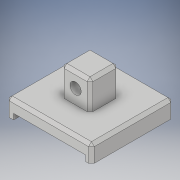
# Autodesk Inventor part: Raspberrycamhalter
Saved by Autodesk Inventor 2018.3 (Build 223284000, 284)
## iProperties
Part Number: Raspberrycamhalter
Material: Generisch
Document SubType Name: Modeling
Designer: pgmadmin
Density: 1 g/cm^3
Appearance: Vorgabe
Author: pgmadmin
Autodesk Inventor part; units mm, degrees
ref_plane "YZ Plane" through (0, 0, 0) normal (1, 0, 0) x (0, 1, 0)
ref_plane "XZ Plane" through (0, 0, 0) normal (0, 1, 0) x (-1, 0, 0)
ref_plane "XY Plane" through (0, 0, 0) normal (0, 0, 1) x (1, 0, 0)
sketch "Skizze1" plane through (0, 0, 0) normal (0, 0, 1) x (1, 0, 0)
  point P0 (0, 0)
sketch "Skizze2" plane through (0, 0, 0) normal (0, 0, 1) x (1, 0, 0)
  line L0 (-12.75, 12.25) -> (12.75, 12.25)
  line L1 (12.75, 12.25) -> (12.75, -12.25)
  line L2 (12.75, -12.25) -> (-12.75, -12.25)
  line L3 (-12.75, -12.25) -> (-12.75, 12.25)
  line L4 (0, 19.95) -> (0, -19.95) projected
  line L5 (-20.65, 0) -> (20.65, 0) projected
  line L6 (-14.75, 14.25) -> (14.75, 14.25)
  line L7 (14.75, 14.25) -> (14.75, -14.25)
  line L8 (14.75, -14.25) -> (-14.75, -14.25)
  line L9 (-14.75, -14.25) -> (-14.75, 14.25)
  point P0 (0, 0)
  dimension "d0" = 25.5
  dimension "d1" = 24.5
  dimension "d2" = 2
  dimension "d3" = 2
  dimension "d4" = 2
  dimension "d5" = 2
  constraints: 16 end point, 4 parallel, 2 horizontal, 2 perpendicular, 2 other
  measures "d0" distance of L1.end L2.end
  measures "d1" distance of L0.end L1.end
  measures "d2" distance between parallel lines of L6 L0
  measures "d3" distance between parallel lines of L3 L9
  measures "d4" distance between parallel lines of L2 L8
  measures "d5" distance between parallel lines of L7 L1
extrude "Extrusion1" add sketch "Skizze2" along normal blind 4 contours L3 L5 L9 L6 L4 L0 | L4 L6 L7 L5 L1 L0 | L3 L2 L4 L8 L9 L5 | L5 L7 L8 L4 L2 L1
sketch "Skizze3" plane through (0, 0, 4) normal (0, 0, 1) x (1, 0, 0)
  line L0 (14.75, -14.25) -> (-14.75, -14.25) projected
  line L1 (-14.75, 14.25) -> (14.75, 14.25)
  line L2 (14.75, 14.25) -> (14.75, -14.25)
  line L3 (14.75, -14.25) -> (-14.75, -14.25)
  line L4 (-14.75, -14.25) -> (-14.75, 14.25)
  point P0 (0, 0)
  constraints: 8 end point, 2 parallel, 1 horizontal, 1 perpendicular
extrude "Extrusion2" add sketch "Skizze3" along normal blind 2
chamfer "Fase1" distance 1 angle 45 8 edges at (14.75, 14.25, 3) (-14.75, 14.25, 3) (-14.75, 0, 6) (0, -14.25, 6) (-14.75, -14.25, 3) (14.75, -14.25, 3) (14.75, 0, 6) (0, 14.25, 6)
sketch "Skizze4" plane through (0, 0, 0) normal (0, 0, -1) x (-1, 0, 0)
  line L0 (12.75, -12.25) -> (-12.75, -12.25) projected
  line L1 (-12.75, -12.25) -> (12.25, -12.25)
  line L2 (12.25, -12.25) -> (12.25, -17.2138)
  line L3 (12.25, -17.2138) -> (-12.75, -17.2138)
  line L4 (-12.75, -17.2138) -> (-12.75, -12.25)
  point P0 (0, 0)
  constraints: 8 end point, 2 parallel, 1 horizontal, 1 perpendicular
extrude "Extrusion3" cut sketch "Skizze4" against normal blind 2
sketch "Skizze5" plane through (0, 0, 0) normal (0, 0, -1) x (-1, 0, 0)
  circle A0 centre (0.25, 13.25) radius 0.5
  line L0 (13.75, 14.25) -> (-13.75, 14.25) projected
  line L1 (14.75, -13.25) -> (14.75, 13.25) projected
  line L2 (-14.75, 13.25) -> (-14.75, -13.25) projected
  circle A1 centre (-9.75, 13.25) radius 0.5
  circle A2 centre (10.25, 13.25) radius 0.5
  circle A3 centre (-13.75, 0.25) radius 0.5
  circle A4 centre (-13.75, -9.75) radius 0.5
  circle A5 centre (-13.75, 10.25) radius 0.5
  line L3 (0, -19.95) -> (0, 19.95) projected
  circle A6 centre (13.75, 0.25) radius 0.5
  circle A7 centre (13.75, -9.75) radius 0.5
  circle A8 centre (13.75, 10.25) radius 0.5
  point P0 (0, 0)
  dimension "d15" = 1
  dimension "d16" = 1
  dimension "d17" = 1
  dimension "d18" = 1
  dimension "d19" = 10
  dimension "d20" = 10
  dimension "d21" = 1
  dimension "d22" = 1
  dimension "d23" = 1
  dimension "d24" = 1
  dimension "d25" = 10
  dimension "d26" = 10
  constraints: 9 centre point, 3 symmetric about line, 3 other
  measures "d15" diameter of A0
  measures "d16" distance from line of L0 A0.centre
  measures "d17" diameter of A1
  measures "d18" diameter of A2
  measures "d19" distance of A0.centre A1.centre
  measures "d20" distance of A2.centre A0.centre
  measures "d21" diameter of A3
  measures "d22" distance from line of L2 A3.centre
  measures "d23" diameter of A4
  measures "d24" diameter of A5
  measures "d25" distance of A3.centre A4.centre
  measures "d26" distance of A3.centre A5.centre
sketch "Skizze6" plane through (0, 0, 6) normal (0, 0, 1) x (1, 0, 0)
  line L0 (-5, 5) -> (5, 5)
  line L1 (5, 5) -> (5, -5)
  line L2 (5, -5) -> (-5, -5)
  line L3 (-5, -5) -> (-5, 5)
  line L4 (0, 19.95) -> (0, -19.95) projected
  line L5 (-20.65, 0) -> (20.65, 0) projected
  point P0 (0, 0)
  dimension "d29" = 10
  dimension "d30" = 10
  constraints: 8 end point, 2 parallel, 1 horizontal, 1 perpendicular, 2 other
  measures "d29" distance of L1.end L2.end
  measures "d30" distance of L0.end L1.end
extrude "Extrusion5" add sketch "Skizze6" along normal blind 10
sketch "Skizze9" plane through (-5, 5, 6) normal (0, 1, 0) x (1, 0, 0)
  circle A0 centre (5, -5) radius 1.95
  line L0 (10, -10) -> (0, -10) projected
  point P0 (5, 6)
  dimension "d52" = 3.9
  dimension "d53" = 5
  constraints: 1 centre point
  measures "d52" diameter of A0
  measures "d53" distance from line of L0 A0.centre
extrude "Extrusion8" cut sketch "Skizze9" against normal blind 26
chamfer "Fase4" distance 1 angle 45 8 edges at (-5, 0, 16) (0, -5, 16) (5, -5, 11) (5, 5, 11) (0, 5, 16) (-5, 5, 11) (-5, -5, 11) (5, 0, 16)
